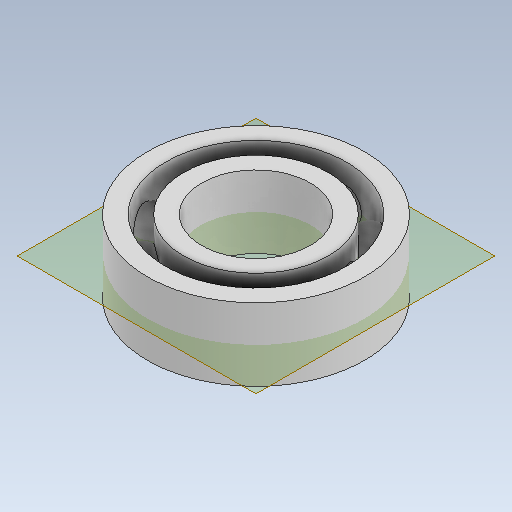
# Autodesk Inventor part: bearing_3_6_2
Saved by Autodesk Inventor 2020 (Build 240168000, 168)
## iProperties
Created: 2020-01-30
Part Number: bearing_3_6_2
Material: Generic
Document SubType Name: Modeling
Designer: psrobotics
Density: 1 g/cm^3
Appearance: Default
Author: psrobotics
Autodesk Inventor part; units mm, degrees
ref_plane "YZ Plane" through (0, 0, 0) normal (1, 0, 0) x (0, 1, 0)
ref_plane "XZ Plane" through (0, 0, 0) normal (0, 1, 0) x (-1, 0, 0)
ref_plane "XY Plane" through (0, 0, 0) normal (0, 0, 1) x (1, 0, 0)
sketch "Sketch1" plane through (0, 0, 0) normal (0, 1, 0) x (-1, 0, 0)
  circle A0 centre (0, 0) radius 3
  circle A1 centre (0, 0) radius 1.5
  dimension "d0" = 6
  dimension "d1" = 3
  constraints: 2 centre point, 2 coincident
  measures "d0" diameter of A0
  measures "d1" diameter of A1
extrude "Extrusion1" add sketch "Sketch1" along normal blind 2
sketch "Sketch2" plane through (0, 0, 0) normal (0, -1, 0) x (1, 0, 0)
  circle A0 centre (0, 0) radius 3 projected
  circle A1 centre (0, 0) radius 1.5 projected
  circle A2 centre (0, 0) radius 2
  circle A3 centre (0, 0) radius 2.5
  dimension "d4" = 4
  dimension "d5" = 5
  constraints: 2 centre point, 2 coincident
  measures "d4" diameter of A2
  measures "d5" diameter of A3
extrude "Extrusion2" cut sketch "Sketch2" against normal blind 2 contours A3
ref_plane "Work Plane1" through (0, 1, 0) normal (0, -1, 0) x (1, 0, 0)
sketch "Sketch3" plane through (0, 1, 0) normal (0, -1, 0) x (1, 0, 0)
  circle A0 centre (0, 0) radius 2 projected
  circle A1 centre (0, 0) radius 2.5 projected
  circle A2 centre (0, 0) radius 2.5 projected
  line L0 (0, 2.5) -> (0, 2)
  circle A3 centre (0, 0) radius 2 projected
  line L1 (0, 2) -> (0, 0)
  circle A4 centre (0, 2.25) radius 0.5
  line L2 (0, 1.75) -> (0, 2.75)
  dimension "d8" = 1
  constraints: 6 end point, 2 point on circle, 2 point on line, 2 vertical, 2 vertical alignment, 1 centre point, 1 midpoint, 2 other
  measures "d8" diameter of A4
revolve "Revolution1" add sketch "Sketch3" angle 360 about axis through (0, 1, 2.5) along (0, 0, -1) picked at (-0.3586, 2.2391) picked at (-0.0845, 1.9198) picked at (-0.0885, 2.5775) contours A4 A1 L0 A0 | A0 L1 A4 | A4 L2 A1
pattern_circular "Circular Pattern1" count 10 over 360 about axis through (0, 0, 0) along (0, 1, 0) of "Revolution1"
body "Solid1"
